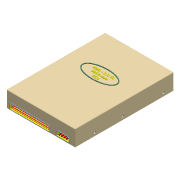
# Autodesk Inventor part: Hdd
Saved by Autodesk Inventor 2016 (Build 200138000, 138)
## iProperties
Created: 2017-12-22
Part Number: Hdd
Material: Generic
Document SubType Name: Modeling
Designer: Adrian
Density: 1 g/cm^3
Appearance: Dark Gray
Author: Adrian
Autodesk Inventor part; units mm, degrees
note: some values were not read from the file. Chosen so that the rebuilt part matches the saved one: offset side.
ref_plane "YZ Plane" through (0, 0, 0) normal (1, 0, 0) x (0, 1, 0)
ref_plane "XZ Plane" through (0, 0, 0) normal (0, 1, 0) x (-1, 0, 0)
ref_plane "XY Plane" through (0, 0, 0) normal (0, 0, 1) x (1, 0, 0)
sketch "Sketch1" plane through (0, 0, 0) normal (0, 0, 1) x (1, 0, 0)
  line L0 (-50.5, -72.5) -> (50.5, -72.5)
  line L1 (50.5, -72.5) -> (50.5, 72.5)
  line L2 (50.5, 72.5) -> (-50.5, 72.5)
  line L3 (-50.5, 72.5) -> (-50.5, -72.5)
  line L4 (0, 101.5) -> (0, -101.5) projected
  line L5 (-70.7, 0) -> (70.7, 0) projected
  dimension "d0" = 101
  dimension "d1" = 145
  dimension "d18" = 50.5
  dimension "d19" = 72.5
  constraints: 8 end point, 2 parallel, 1 horizontal, 1 perpendicular
  measures "d0" distance of L2.end L1.end
  measures "d1" distance of L1.end L0.end
  measures "d18" distance between parallel lines of L1 L4
  measures "d19" distance between parallel lines of L5 L2
extrude "Extrusion1" add sketch "Sketch1" along normal blind 24
fillet "Fillet1" radius 1 4 edges at (0, -72.5, 24) (50.5, 0, 24) (0, 72.5, 24) (-50.5, 0, 24)
fillet "Fillet2" radius 1 4 edges at (0, -72.5, 0) (-50.5, 0, 0) (0, 72.5, 0) (50.5, 0, 0)
fillet "Fillet3" radius 1 12 edges at (-50.2071, 72.2071, 23.7071) (-50.2071, 72.2071, 0.2929) (-50.5, 72.5, 12) (-50.2071, -72.2071, 23.7071) (-50.2071, -72.2071, 0.2929) (-50.5, -72.5, 12) (50.2071, -72.2071, 23.7071) (50.2071, -72.2071, 0.2929) (50.5, -72.5, 12) (50.2071, 72.2071, 23.7071) (50.2071, 72.2071, 0.2929) (50.5, 72.5, 12)
sketch "Sketch2" plane through (-50.5, -71.5, 23) normal (-1, 0, 0) x (0, 0, 1)
  line L0 (-23, 143) -> (-23, 0) projected
  line L1 (0, 144) -> (-22, 144) projected
  point P0 (-18, 129)
  point P1 (-18, 69)
  point P2 (-18, 28)
  dimension "d7" = 5
  dimension "d8" = 15
  dimension "d9" = 60
  dimension "d10" = 41
  constraints: 2 vertical alignment
  measures "d7" distance from line of L0 point (-18, 28)
  measures "d8" distance from line of L1 point (-18, 129)
  measures "d9" distance of point (-18, 129) point (-18, 69)
  measures "d10" distance of point (-18, 28) point (-18, 69)
hole "Hole1" at (-50.5, 57.5, 5) at (-50.5, -2.5, 5) at (-50.5, -43.5, 5) direction (1, 0, 0) diameter 3.242 depth 11.8 tip angle 118 thread size "M4x0.7" class "6H" standard "ISO Metric profile"
mirror "Mirror1" about plane through (0, 0, 0) normal (1, 0, 0) of "Hole1"
sketch "Sketch3" plane through (-49.5, -72.5, 23) normal (0, -1, 0) x (1, 0, 0)
  line L0 (4.4644, -13.9434) -> (62.4644, -13.9434)
  line L1 (62.4644, -13.9434) -> (62.4644, -20.9434)
  line L2 (62.4644, -20.9434) -> (4.4644, -20.9434)
  line L3 (4.4644, -20.9434) -> (4.4644, -13.9434)
  dimension "d20" = 7
  dimension "d21" = 58
  constraints: 8 end point, 2 parallel, 1 horizontal, 1 perpendicular
  measures "d20" distance of L2.end L0.start
  measures "d21" distance of L0.start L0.end
extrude "Extrusion2" cut sketch "Sketch3" against normal blind 8
sketch "Sketch4" plane through (-49.5, -64.5, 23) normal (0, -1, 0) x (1, 0, 0)
  line L0 (4.4644, -13.9434) -> (62.4644, -13.9434) projected
  line L1 (4.4644, -20.9434) -> (4.4644, -13.9434) projected
  circle A0 centre (7.0044, -16.4834) radius 0.5
  dimension "d26" = 2.54
  dimension "d27" = 2.54
  dimension "d34" = 1
  constraints: 1 centre point, 1 coincident
  measures "d26" distance from line of L0 point (7.004, -16.483)
  measures "d27" distance from line of L1 point (7.004, -16.483)
  measures "d34" diameter of A0
extrude "Extrusion3" add sketch "Sketch4" along normal blind 8
pattern_linear "Rectangular Pattern2" count 24 spacing 2.54 along (1, 0, 0) count 2 spacing 2.54 along (0, 0, -1) of "Extrusion3"
sketch "Sketch5" plane through (0, 0, 24) normal (0, 0, 1) x (1, 0, 0)
  line L0 (-19.8246, 19.2815) -> (19.8246, 19.2815) construction
  line L1 (19.8246, 19.2815) -> (19.8246, 9.0193) construction
  line L2 (19.8246, 9.0193) -> (-19.8246, 9.0193) construction
  line L3 (-19.8246, 9.0193) -> (-19.8246, 19.2815) construction
  line L4 (49.5, 72.5) -> (-49.5, 72.5) construction
  line L5 (-12.1323, 18.1219) -> (-13.0115, 18.1219)
  line L6 (-13.0115, 18.1219) -> (-13.0115, 19.6734)
  line L7 (-13.0115, 19.6734) -> (-14.2056, 19.6734)
  line L8 (-14.2056, 19.6734) -> (-14.2056, 18.1219)
  line L9 (-14.2056, 18.1219) -> (-15.0849, 18.1219)
  line L10 (-15.0849, 18.1219) -> (-15.0849, 21.6219)
  line L11 (-15.0849, 21.6219) -> (-14.2056, 21.6219)
  line L12 (-14.2056, 21.6219) -> (-14.2056, 20.3399)
  line L13 (-14.2056, 20.3399) -> (-13.0115, 20.3399)
  line L14 (-13.0115, 20.3399) -> (-13.0115, 21.6219)
  line L15 (-13.0115, 21.6219) -> (-12.1323, 21.6219)
  line L16 (-12.1323, 21.6219) -> (-12.1323, 18.1219)
  spline S0 degree 2 poles (-8.2834, 19.8691) (-8.2834, 19.3784) (-8.7117, 18.6069) (-9.0379, 18.3999) knots 0 0 0 1 2 2 2
  spline S1 degree 2 poles (-9.0379, 18.3999) (-9.3102, 18.224) (-9.9512, 18.1219) (-10.3114, 18.1219) knots 0 0 0 1 2 2 2
  line L17 (-10.3114, 18.1219) -> (-11.4062, 18.1219)
  line L18 (-11.4062, 18.1219) -> (-11.4062, 21.6219)
  line L19 (-11.4062, 21.6219) -> (-10.3227, 21.6219)
  spline S2 degree 2 poles (-10.3227, 21.6219) (-9.954, 21.6219) (-9.3102, 21.5283) (-9.0265, 21.3468) knots 0 0 0 1 2 2 2
  spline S3 degree 2 poles (-9.0265, 21.3468) (-8.6833, 21.1256) (-8.2834, 20.3768) (-8.2834, 19.8691) knots 0 0 0 1 2 2 2
  spline S4 degree 2 poles (-9.1854, 19.8747) (-9.1854, 20.2208) (-9.4236, 20.7143) (-9.6675, 20.8533) knots 0 0 0 1 2 2 2
  spline S5 degree 2 poles (-9.6675, 20.8533) (-9.8462, 20.9497) (-10.2376, 20.9696) (-10.5099, 20.9696) knots 0 0 0 1 2 2 2
  line L20 (-10.5099, 20.9696) -> (-10.5269, 20.9696)
  line L21 (-10.5269, 20.9696) -> (-10.5269, 18.7771)
  line L22 (-10.5269, 18.7771) -> (-10.5099, 18.7771)
  spline S6 degree 2 poles (-10.5099, 18.7771) (-10.215, 18.7771) (-9.8094, 18.7969) (-9.625, 18.9132) knots 0 0 0 1 2 2 2
  spline S7 degree 2 poles (-9.625, 18.9132) (-9.4094, 19.0494) (-9.1854, 19.5287) (-9.1854, 19.8747) knots 0 0 0 1 2 2 2
  spline S8 degree 2 poles (-4.6388, 19.8691) (-4.6388, 19.3784) (-5.0671, 18.6069) (-5.3932, 18.3999) knots 0 0 0 1 2 2 2
  spline S9 degree 2 poles (-5.3932, 18.3999) (-5.6655, 18.224) (-6.3065, 18.1219) (-6.6667, 18.1219) knots 0 0 0 1 2 2 2
  line L23 (-6.6667, 18.1219) -> (-7.7615, 18.1219)
  line L24 (-7.7615, 18.1219) -> (-7.7615, 21.6219)
  line L25 (-7.7615, 21.6219) -> (-6.6781, 21.6219)
  spline S10 degree 2 poles (-6.6781, 21.6219) (-6.3094, 21.6219) (-5.6655, 21.5283) (-5.3819, 21.3468) knots 0 0 0 1 2 2 2
  spline S11 degree 2 poles (-5.3819, 21.3468) (-5.0387, 21.1256) (-4.6388, 20.3768) (-4.6388, 19.8691) knots 0 0 0 1 2 2 2
  spline S12 degree 2 poles (-5.5407, 19.8747) (-5.5407, 20.2208) (-5.779, 20.7143) (-6.0229, 20.8533) knots 0 0 0 1 2 2 2
  spline S13 degree 2 poles (-6.0229, 20.8533) (-6.2016, 20.9497) (-6.593, 20.9696) (-6.8653, 20.9696) knots 0 0 0 1 2 2 2
  line L26 (-6.8653, 20.9696) -> (-6.8823, 20.9696)
  line L27 (-6.8823, 20.9696) -> (-6.8823, 18.7771)
  line L28 (-6.8823, 18.7771) -> (-6.8653, 18.7771)
  spline S14 degree 2 poles (-6.8653, 18.7771) (-6.5703, 18.7771) (-6.1647, 18.7969) (-5.9803, 18.9132) knots 0 0 0 1 2 2 2
  spline S15 degree 2 poles (-5.9803, 18.9132) (-5.7648, 19.0494) (-5.5407, 19.5287) (-5.5407, 19.8747) knots 0 0 0 1 2 2 2
  line L29 (-1.2551, 19.3415) -> (-2.8122, 19.3415)
  line L30 (-2.8122, 19.3415) -> (-2.8122, 19.9939)
  line L31 (-2.8122, 19.9939) -> (-1.2551, 19.9939)
  line L32 (-1.2551, 19.9939) -> (-1.2551, 19.3415)
  line L33 (3.1866, 18.1219) -> (0.875, 18.1219)
  line L34 (0.875, 18.1219) -> (0.875, 18.7317)
  line L35 (0.875, 18.7317) -> (1.6124, 18.7317)
  line L36 (1.6124, 18.7317) -> (1.6124, 20.5838)
  line L37 (1.6124, 20.5838) -> (0.875, 20.5838)
  line L38 (0.875, 20.5838) -> (0.875, 21.1539)
  spline S16 degree 2 poles (0.875, 21.1539) (1.0367, 21.1539) (1.3572, 21.1965) (1.4536, 21.2418) knots 0 0 0 1 2 2 2
  spline S17 degree 2 poles (1.4536, 21.2418) (1.5642, 21.2986) (1.689, 21.4886) (1.7004, 21.6304) knots 0 0 0 1 2 2 2
  line L39 (1.7004, 21.6304) -> (2.4662, 21.6304)
  line L40 (2.4662, 21.6304) -> (2.4662, 18.7317)
  line L41 (2.4662, 18.7317) -> (3.1866, 18.7317)
  line L42 (3.1866, 18.7317) -> (3.1866, 18.1219)
  line L43 (4.6473, 18.1219) -> (3.8162, 18.1219)
  line L44 (3.8162, 18.1219) -> (3.8162, 19.0465)
  line L45 (3.8162, 19.0465) -> (4.6473, 19.0465)
  line L46 (4.6473, 19.0465) -> (4.6473, 18.1219)
  spline S18 degree 2 poles (7.8665, 19.8719) (7.8665, 19.4181) (7.7218, 18.7374) (7.5602, 18.5076) knots 0 0 0 1 2 2 2
  spline S19 degree 2 poles (7.5602, 18.5076) (7.4013, 18.2807) (6.888, 18.0482) (6.5192, 18.0482) knots 0 0 0 1 2 2 2
  spline S20 degree 2 poles (6.5192, 18.0482) (6.1477, 18.0482) (5.6372, 18.2807) (5.4755, 18.5133) knots 0 0 0 1 2 2 2
  spline S21 degree 2 poles (5.4755, 18.5133) (5.3138, 18.7431) (5.1692, 19.4181) (5.1692, 19.8719) knots 0 0 0 1 2 2 2
  spline S22 degree 2 poles (5.1692, 19.8719) (5.1692, 20.3371) (5.3138, 20.9951) (5.4783, 21.2333) knots 0 0 0 1 2 2 2
  spline S23 degree 2 poles (5.4783, 21.2333) (5.6428, 21.4659) (6.1619, 21.6928) (6.5192, 21.6928) knots 0 0 0 1 2 2 2
  spline S24 degree 2 poles (6.5192, 21.6928) (6.8965, 21.6928) (7.4013, 21.4546) (7.563, 21.2192) knots 0 0 0 1 2 2 2
  spline S25 degree 2 poles (7.563, 21.2192) (7.7218, 20.9894) (7.8665, 20.3115) (7.8665, 19.8719) knots 0 0 0 1 2 2 2
  spline S26 degree 2 poles (6.9844, 19.8719) (6.9844, 20.5214) (6.7717, 21.0461) (6.5192, 21.0461) knots 0 0 0 1 2 2 2
  spline S27 degree 2 poles (6.5192, 21.0461) (6.2668, 21.0461) (6.0513, 20.5214) (6.0513, 19.8691) knots 0 0 0 1 2 2 2
  spline S28 degree 2 poles (6.0513, 19.8691) (6.0513, 19.2281) (6.2668, 18.6948) (6.5192, 18.6948) knots 0 0 0 1 2 2 2
  spline S29 degree 2 poles (6.5192, 18.6948) (6.7688, 18.6948) (6.9844, 19.2281) (6.9844, 19.8719) knots 0 0 0 1 2 2 2
  line L47 (10.4957, 18.1219) -> (10.4957, 20.9554)
  line L48 (10.4957, 20.9554) -> (9.4605, 20.9554)
  line L49 (9.4605, 20.9554) -> (9.4605, 21.6219)
  line L50 (9.4605, 21.6219) -> (12.4103, 21.6219)
  line L51 (12.4103, 21.6219) -> (12.4103, 20.9554)
  line L52 (12.4103, 20.9554) -> (11.375, 20.9554)
  line L53 (11.375, 20.9554) -> (11.375, 18.1219)
  line L54 (11.375, 18.1219) -> (10.4957, 18.1219)
  spline S30 degree 2 poles (15.309, 19.4777) (15.309, 18.848) (14.6708, 18.0709) (14.1971, 18.0709) knots 0 0 0 1 2 2 2
  spline S31 degree 2 poles (14.1971, 18.0709) (14.0014, 18.0709) (13.7093, 18.1588) (13.5448, 18.2524) knots 0 0 0 1 2 2 2
  line L55 (13.5448, 18.2524) -> (13.5107, 18.1219)
  line L56 (13.5107, 18.1219) -> (12.7222, 18.1219)
  line L57 (12.7222, 18.1219) -> (12.7222, 21.7779)
  line L58 (12.7222, 21.7779) -> (13.5448, 21.7779)
  line L59 (13.5448, 21.7779) -> (13.5448, 20.4845)
  spline S32 degree 2 poles (13.5448, 20.4845) (13.7263, 20.6405) (14.1007, 20.8334) (14.3474, 20.8334) knots 0 0 0 1 2 2 2
  spline S33 degree 2 poles (14.3474, 20.8334) (14.8098, 20.8334) (15.309, 20.1158) (15.309, 19.4777) knots 0 0 0 1 2 2 2
  spline S34 degree 2 poles (14.4666, 19.4606) (14.4666, 19.8549) (14.2283, 20.1924) (13.9787, 20.1924) knots 0 0 0 1 2 2 2
  spline S35 degree 2 poles (13.9787, 20.1924) (13.8681, 20.1924) (13.6497, 20.1215) (13.5448, 20.0506) knots 0 0 0 1 2 2 2
  line L60 (13.5448, 20.0506) -> (13.5448, 18.7289)
  spline S36 degree 2 poles (13.5448, 18.7289) (13.627, 18.6948) (13.7944, 18.6721) (13.8766, 18.6721) knots 0 0 0 1 2 2 2
  spline S37 degree 2 poles (13.8766, 18.6721) (14.1744, 18.6721) (14.4666, 19.0664) (14.4666, 19.4606) knots 0 0 0 1 2 2 2
  line L61 (-8.8393, 15.1644) -> (-10.3341, 12.3592)
  line L62 (-10.3341, 12.3592) -> (-11.3098, 12.3592)
  line L63 (-11.3098, 12.3592) -> (-9.747, 15.1984)
  line L64 (-9.747, 15.1984) -> (-11.4147, 15.1984)
  line L65 (-11.4147, 15.1984) -> (-11.4147, 15.8592)
  line L66 (-11.4147, 15.8592) -> (-8.8393, 15.8592)
  line L67 (-8.8393, 15.8592) -> (-8.8393, 15.1644)
  line L68 (-5.6967, 12.3592) -> (-8.2692, 12.3592)
  line L69 (-8.2692, 12.3592) -> (-8.2692, 12.9293)
  spline S38 degree 2 poles (-8.2692, 12.9293) (-7.9431, 13.1903) (-7.4212, 13.6498) (-7.2255, 13.8568) knots 0 0 0 1 2 2 2
  spline S39 degree 2 poles (-7.2255, 13.8568) (-6.9674, 14.1263) (-6.7376, 14.5375) (-6.7376, 14.7531) knots 0 0 0 1 2 2 2
  spline S40 degree 2 poles (-6.7376, 14.7531) (-6.7376, 14.997) (-7.0298, 15.258) (-7.2907, 15.258) knots 0 0 0 1 2 2 2
  spline S41 degree 2 poles (-7.2907, 15.258) (-7.424, 15.258) (-7.6623, 15.1927) (-7.7842, 15.1417) knots 0 0 0 1 2 2 2
  spline S42 degree 2 poles (-7.7842, 15.1417) (-7.9034, 15.0878) (-8.0735, 14.9743) (-8.1161, 14.946) knots 0 0 0 1 2 2 2
  line L70 (-8.1161, 14.946) -> (-8.1842, 14.946)
  line L71 (-8.1842, 14.946) -> (-8.1842, 15.7089)
  spline S43 degree 2 poles (-8.1842, 15.7089) (-8.0367, 15.7798) (-7.407, 15.9273) (-7.1149, 15.9273) knots 0 0 0 1 2 2 2
  spline S44 degree 2 poles (-7.1149, 15.9273) (-6.4909, 15.9273) (-5.8499, 15.3714) (-5.8499, 14.8694) knots 0 0 0 1 2 2 2
  spline S45 degree 2 poles (-5.8499, 14.8694) (-5.8499, 14.5602) (-6.142, 13.9646) (-6.4795, 13.6242) knots 0 0 0 1 2 2 2
  spline S46 degree 2 poles (-6.4795, 13.6242) (-6.6923, 13.4144) (-7.0922, 13.0882) (-7.1801, 13.0201) knots 0 0 0 1 2 2 2
  line L72 (-7.1801, 13.0201) -> (-5.6967, 13.0201)
  line L73 (-5.6967, 13.0201) -> (-5.6967, 12.3592)
  spline S47 degree 2 poles (-2.6761, 14.1092) (-2.6761, 13.6554) (-2.8207, 12.9747) (-2.9824, 12.745) knots 0 0 0 1 2 2 2
  spline S48 degree 2 poles (-2.9824, 12.745) (-3.1412, 12.5181) (-3.6546, 12.2855) (-4.0233, 12.2855) knots 0 0 0 1 2 2 2
  spline S49 degree 2 poles (-4.0233, 12.2855) (-4.3949, 12.2855) (-4.9054, 12.5181) (-5.0671, 12.7507) knots 0 0 0 1 2 2 2
  spline S50 degree 2 poles (-5.0671, 12.7507) (-5.2287, 12.9804) (-5.3734, 13.6554) (-5.3734, 14.1092) knots 0 0 0 1 2 2 2
  spline S51 degree 2 poles (-5.3734, 14.1092) (-5.3734, 14.5744) (-5.2287, 15.2324) (-5.0642, 15.4707) knots 0 0 0 1 2 2 2
  spline S52 degree 2 poles (-5.0642, 15.4707) (-4.8997, 15.7033) (-4.3807, 15.9302) (-4.0233, 15.9302) knots 0 0 0 1 2 2 2
  spline S53 degree 2 poles (-4.0233, 15.9302) (-3.6461, 15.9302) (-3.1412, 15.6919) (-2.9795, 15.4565) knots 0 0 0 1 2 2 2
  spline S54 degree 2 poles (-2.9795, 15.4565) (-2.8207, 15.2268) (-2.6761, 14.5489) (-2.6761, 14.1092) knots 0 0 0 1 2 2 2
  spline S55 degree 2 poles (-3.5581, 14.1092) (-3.5581, 14.7588) (-3.7709, 15.2835) (-4.0233, 15.2835) knots 0 0 0 1 2 2 2
  spline S56 degree 2 poles (-4.0233, 15.2835) (-4.2757, 15.2835) (-4.4913, 14.7588) (-4.4913, 14.1064) knots 0 0 0 1 2 2 2
  spline S57 degree 2 poles (-4.4913, 14.1064) (-4.4913, 13.4654) (-4.2757, 12.9322) (-4.0233, 12.9322) knots 0 0 0 1 2 2 2
  spline S58 degree 2 poles (-4.0233, 12.9322) (-3.7737, 12.9322) (-3.5581, 13.4654) (-3.5581, 14.1092) knots 0 0 0 1 2 2 2
  spline S59 degree 2 poles (0.39, 14.1092) (0.39, 13.6554) (0.2453, 12.9747) (0.0837, 12.745) knots 0 0 0 1 2 2 2
  spline S60 degree 2 poles (0.0837, 12.745) (-0.0752, 12.5181) (-0.5885, 12.2855) (-0.9573, 12.2855) knots 0 0 0 1 2 2 2
  spline S61 degree 2 poles (-0.9573, 12.2855) (-1.3288, 12.2855) (-1.8393, 12.5181) (-2.001, 12.7507) knots 0 0 0 1 2 2 2
  spline S62 degree 2 poles (-2.001, 12.7507) (-2.1627, 12.9804) (-2.3073, 13.6554) (-2.3073, 14.1092) knots 0 0 0 1 2 2 2
  spline S63 degree 2 poles (-2.3073, 14.1092) (-2.3073, 14.5744) (-2.1627, 15.2324) (-1.9982, 15.4707) knots 0 0 0 1 2 2 2
  spline S64 degree 2 poles (-1.9982, 15.4707) (-1.8337, 15.7033) (-1.3146, 15.9302) (-0.9573, 15.9302) knots 0 0 0 1 2 2 2
  spline S65 degree 2 poles (-0.9573, 15.9302) (-0.58, 15.9302) (-0.0752, 15.6919) (0.0865, 15.4565) knots 0 0 0 1 2 2 2
  spline S66 degree 2 poles (0.0865, 15.4565) (0.2453, 15.2268) (0.39, 14.5489) (0.39, 14.1092) knots 0 0 0 1 2 2 2
  spline S67 degree 2 poles (-0.4921, 14.1092) (-0.4921, 14.7588) (-0.7048, 15.2835) (-0.9573, 15.2835) knots 0 0 0 1 2 2 2
  spline S68 degree 2 poles (-0.9573, 15.2835) (-1.2097, 15.2835) (-1.4252, 14.7588) (-1.4252, 14.1064) knots 0 0 0 1 2 2 2
  spline S69 degree 2 poles (-1.4252, 14.1064) (-1.4252, 13.4654) (-1.2097, 12.9322) (-0.9573, 12.9322) knots 0 0 0 1 2 2 2
  spline S70 degree 2 poles (-0.9573, 12.9322) (-0.7077, 12.9322) (-0.4921, 13.4654) (-0.4921, 14.1092) knots 0 0 0 1 2 2 2
  line L74 (4.0715, 14.2199) -> (4.0034, 14.2199)
  spline S71 degree 2 poles (4.0034, 14.2199) (3.9552, 14.2369) (3.7765, 14.2539) (3.6688, 14.2539) knots 0 0 0 1 2 2 2
  spline S72 degree 2 poles (3.6688, 14.2539) (3.5411, 14.2539) (3.2547, 14.1773) (3.1214, 14.1263) knots 0 0 0 1 2 2 2
  line L75 (3.1214, 14.1263) -> (3.1214, 12.3592)
  line L76 (3.1214, 12.3592) -> (2.2988, 12.3592)
  line L77 (2.2988, 12.3592) -> (2.2988, 14.9998)
  line L78 (2.2988, 14.9998) -> (3.1214, 14.9998)
  line L79 (3.1214, 14.9998) -> (3.1214, 14.6198)
  spline S73 degree 2 poles (3.1214, 14.6198) (3.1781, 14.6708) (3.3766, 14.8297) (3.4589, 14.8779) knots 0 0 0 1 2 2 2
  spline S74 degree 2 poles (3.4589, 14.8779) (3.5496, 14.9318) (3.7879, 15.0084) (3.8928, 15.0084) knots 0 0 0 1 2 2 2
  spline S75 degree 2 poles (3.8928, 15.0084) (3.9325, 15.0084) (4.0318, 15.0027) (4.0715, 14.9998) knots 0 0 0 1 2 2 2
  line L80 (4.0715, 14.9998) -> (4.0715, 14.2199)
  spline S76 degree 2 poles (6.9731, 13.715) (6.9731, 13.0825) (6.332, 12.3082) (5.8612, 12.3082) knots 0 0 0 1 2 2 2
  spline S77 degree 2 poles (5.8612, 12.3082) (5.6655, 12.3082) (5.3734, 12.3961) (5.2089, 12.4926) knots 0 0 0 1 2 2 2
  line L81 (5.2089, 12.4926) -> (5.2089, 11.3921)
  line L82 (5.2089, 11.3921) -> (4.3863, 11.3921)
  line L83 (4.3863, 11.3921) -> (4.3863, 14.9998)
  line L84 (4.3863, 14.9998) -> (5.2089, 14.9998)
  line L85 (5.2089, 14.9998) -> (5.2089, 14.7219)
  spline S78 degree 2 poles (5.2089, 14.7219) (5.3904, 14.8779) (5.7648, 15.0708) (6.0115, 15.0708) knots 0 0 0 1 2 2 2
  spline S79 degree 2 poles (6.0115, 15.0708) (6.471, 15.0708) (6.9731, 14.3418) (6.9731, 13.715) knots 0 0 0 1 2 2 2
  spline S80 degree 2 poles (6.1307, 13.698) (6.1307, 14.0837) (5.8924, 14.4298) (5.6428, 14.4298) knots 0 0 0 1 2 2 2
  spline S81 degree 2 poles (5.6428, 14.4298) (5.5322, 14.4298) (5.3138, 14.3588) (5.2089, 14.2879) knots 0 0 0 1 2 2 2
  line L86 (5.2089, 14.2879) -> (5.2089, 12.9634)
  spline S82 degree 2 poles (5.2089, 12.9634) (5.2741, 12.935) (5.4329, 12.9123) (5.5407, 12.9123) knots 0 0 0 1 2 2 2
  spline S83 degree 2 poles (5.5407, 12.9123) (5.8385, 12.9123) (6.1307, 13.3037) (6.1307, 13.698) knots 0 0 0 1 2 2 2
  line L87 (10.5667, 12.3592) -> (10.5667, 13.6781)
  spline S84 degree 2 poles (10.5667, 13.6781) (10.5667, 13.8738) (10.5525, 14.1404) (10.5184, 14.2255) knots 0 0 0 1 2 2 2
  spline S85 degree 2 poles (10.5184, 14.2255) (10.4816, 14.3106) (10.3341, 14.3872) (10.2008, 14.3872) knots 0 0 0 1 2 2 2
  spline S86 degree 2 poles (10.2008, 14.3872) (10.1072, 14.3872) (9.9256, 14.305) (9.8179, 14.2284) knots 0 0 0 1 2 2 2
  line L88 (9.8179, 14.2284) -> (9.8179, 12.3592)
  line L89 (9.8179, 12.3592) -> (8.9897, 12.3592)
  line L90 (8.9897, 12.3592) -> (8.9897, 13.6781)
  spline S87 degree 2 poles (8.9897, 13.6781) (8.9897, 13.871) (8.9726, 14.1404) (8.9386, 14.2255) knots 0 0 0 1 2 2 2
  spline S88 degree 2 poles (8.9386, 14.2255) (8.9017, 14.3106) (8.7543, 14.3872) (8.6209, 14.3872) knots 0 0 0 1 2 2 2
  spline S89 degree 2 poles (8.6209, 14.3872) (8.5217, 14.3872) (8.326, 14.2936) (8.2352, 14.2284) knots 0 0 0 1 2 2 2
  line L91 (8.2352, 14.2284) -> (8.2352, 12.3592)
  line L92 (8.2352, 12.3592) -> (7.4127, 12.3592)
  line L93 (7.4127, 12.3592) -> (7.4127, 14.9998)
  line L94 (7.4127, 14.9998) -> (8.2352, 14.9998)
  line L95 (8.2352, 14.9998) -> (8.2352, 14.7077)
  spline S90 degree 2 poles (8.2352, 14.7077) (8.4366, 14.8779) (8.7968, 15.0708) (9.0209, 15.0708) knots 0 0 0 1 2 2 2
  spline S91 degree 2 poles (9.0209, 15.0708) (9.262, 15.0708) (9.6307, 14.841) (9.7271, 14.6113) knots 0 0 0 1 2 2 2
  spline S92 degree 2 poles (9.7271, 14.6113) (9.9625, 14.8325) (10.3823, 15.0708) (10.5979, 15.0708) knots 0 0 0 1 2 2 2
  spline S93 degree 2 poles (10.5979, 15.0708) (10.7822, 15.0708) (11.0744, 14.9545) (11.1736, 14.8353) knots 0 0 0 1 2 2 2
  spline S94 degree 2 poles (11.1736, 14.8353) (11.2842, 14.7077) (11.3949, 14.3588) (11.3949, 14.078) knots 0 0 0 1 2 2 2
  line L96 (11.3949, 14.078) -> (11.3949, 12.3592)
  line L97 (11.3949, 12.3592) -> (10.5667, 12.3592)
  spline S95 degree 2 poles (-2.9994, 6.5228) (-3.7056, 6.5228) (-4.4658, 7.2036) (-4.4658, 7.8616) knots 0 0 0 1 2 2 2
  line L98 (-4.4658, 7.8616) -> (-4.4658, 10.0966)
  line L99 (-4.4658, 10.0966) -> (-3.5865, 10.0966)
  line L100 (-3.5865, 10.0966) -> (-3.5865, 7.9126)
  spline S96 degree 2 poles (-3.5865, 7.9126) (-3.5865, 7.5468) (-3.3114, 7.1894) (-2.9994, 7.1894) knots 0 0 0 1 2 2 2
  spline S97 degree 2 poles (-2.9994, 7.1894) (-2.6959, 7.1894) (-2.4123, 7.5326) (-2.4123, 7.9126) knots 0 0 0 1 2 2 2
  line L101 (-2.4123, 7.9126) -> (-2.4123, 10.0966)
  line L102 (-2.4123, 10.0966) -> (-1.533, 10.0966)
  line L103 (-1.533, 10.0966) -> (-1.533, 7.8644)
  spline S98 degree 2 poles (-1.533, 7.8644) (-1.533, 7.2177) (-2.2733, 6.5228) (-2.9994, 6.5228) knots 0 0 0 1 2 2 2
  spline S99 degree 2 poles (0.6509, 6.5285) (-0.1376, 6.5285) (-1.0622, 7.4815) (-1.0622, 8.3438) knots 0 0 0 1 2 2 2
  spline S100 degree 2 poles (-1.0622, 8.3438) (-1.0622, 9.1748) (-0.1347, 10.1647) (0.6538, 10.1647) knots 0 0 0 1 2 2 2
  spline S101 degree 2 poles (0.6538, 10.1647) (0.8608, 10.1647) (1.1955, 10.1164) (1.3487, 10.0767) knots 0 0 0 1 2 2 2
  spline S102 degree 2 poles (1.3487, 10.0767) (1.4678, 10.0399) (1.7486, 9.9179) (1.8365, 9.8725) knots 0 0 0 1 2 2 2
  line L104 (1.8365, 9.8725) -> (1.8365, 9.0386)
  line L105 (1.8365, 9.0386) -> (1.7486, 9.0386)
  spline S103 degree 2 poles (1.7486, 9.0386) (1.6833, 9.0954) (1.4905, 9.2542) (1.3685, 9.328) knots 0 0 0 1 2 2 2
  spline S104 degree 2 poles (1.3685, 9.328) (1.2466, 9.4045) (0.9544, 9.5095) (0.7927, 9.5095) knots 0 0 0 1 2 2 2
  spline S105 degree 2 poles (0.7927, 9.5095) (0.6027, 9.5095) (0.2879, 9.3904) (0.1432, 9.24) knots 0 0 0 1 2 2 2
  spline S106 degree 2 poles (0.1432, 9.24) (0.0128, 9.1067) (-0.1546, 8.6501) (-0.1546, 8.3409) knots 0 0 0 1 2 2 2
  spline S107 degree 2 poles (-0.1546, 8.3409) (-0.1546, 8.0147) (0.0184, 7.5694) (0.1603, 7.4333) knots 0 0 0 1 2 2 2
  spline S108 degree 2 poles (0.1603, 7.4333) (0.2964, 7.3) (0.6311, 7.1837) (0.7984, 7.1837) knots 0 0 0 1 2 2 2
  spline S109 degree 2 poles (0.7984, 7.1837) (0.9714, 7.1837) (1.2863, 7.3) (1.394, 7.3709) knots 0 0 0 1 2 2 2
  spline S110 degree 2 poles (1.394, 7.3709) (1.5132, 7.4418) (1.6919, 7.5921) (1.7571, 7.6517) knots 0 0 0 1 2 2 2
  line L106 (1.7571, 7.6517) -> (1.8365, 7.6517)
  line L107 (1.8365, 7.6517) -> (1.8365, 6.8292)
  spline S111 degree 2 poles (1.8365, 6.8292) (1.7401, 6.7838) (1.4876, 6.6703) (1.3515, 6.6306) knots 0 0 0 1 2 2 2
  spline S112 degree 2 poles (1.3515, 6.6306) (1.187, 6.5796) (0.9005, 6.5285) (0.6509, 6.5285) knots 0 0 0 1 2 2 2
  line L108 (4.7778, 9.2372) -> (3.8304, 6.5966)
  line L109 (3.8304, 6.5966) -> (2.9313, 6.5966)
  line L110 (2.9313, 6.5966) -> (1.9925, 9.2372)
  line L111 (1.9925, 9.2372) -> (2.8576, 9.2372)
  line L112 (2.8576, 9.2372) -> (3.3965, 7.4929)
  line L113 (3.3965, 7.4929) -> (3.9297, 9.2372)
  line L114 (3.9297, 9.2372) -> (4.7778, 9.2372)
  point P0 (0, 19.2815)
  point P1 (0, 72.5)
  constraints: 2 midpoint, 1 vertical alignment, 2 other
sketch "Sketch6" plane through (-49.5, -72.5, 23) normal (0, -1, 0) x (1, 0, 0)
  line L0 (73, -16.5) -> (73, -20.5)
  line L1 (73, -20.5) -> (91, -20.5)
  line L2 (91, -20.5) -> (91, -16.5)
  line L3 (91, -16.5) -> (89, -14.5)
  line L4 (89, -14.5) -> (75, -14.5)
  line L5 (75, -14.5) -> (73, -16.5)
  line L6 (0, -23) -> (99, -23) projected
  line L7 (100, -22) -> (100, 0) projected
  dimension "d43" = 18
  dimension "d44" = 6
  dimension "d45" = 2.5
  dimension "d46" = 9
  dimension "d47" = 14
  constraints: 12 end point, 3 perpendicular, 2 equal length, 1 parallel, 1 vertical
  measures "d43" distance of L0.end L1.end
  measures "d44" distance between parallel lines of L1 L4
  measures "d45" distance between parallel lines of L6 L1
  measures "d46" distance between parallel lines of L7 L2
  measures "d47" distance of L3.end L4.end
extrude "Extrusion4" cut sketch "Sketch6" against normal blind 8
sketch "Sketch7" plane through (-49.5, -64.5, 23) normal (0, -1, 0) x (1, 0, 0)
  circle A0 centre (76.5, -18.1) radius 1
  line L0 (91, -20.5) -> (73, -20.5) projected
  circle A1 centre (80, -18.1) radius 1
  circle A2 centre (83.5, -18.1) radius 1
  circle A3 centre (87, -18.1) radius 1
  line L1 (73, -20.5) -> (73, -16.5) projected
  dimension "d50" = 2
  dimension "d51" = 2.4
  dimension "d52" = 2
  dimension "d53" = 2
  dimension "d54" = 2
  dimension "d55" = 3.5
  dimension "d56" = 3.5
  dimension "d57" = 3.5
  dimension "d58" = 3.5
  constraints: 4 centre point, 3 horizontal alignment
  measures "d50" diameter of A0
  measures "d51" distance from line of A0.centre L0
  measures "d52" diameter of A1
  measures "d53" diameter of A2
  measures "d54" diameter of A3
  measures "d55" distance of A1.centre A0.centre
  measures "d56" distance of A2.centre A1.centre
  measures "d57" distance of A2.centre A3.centre
  measures "d58" distance from line of L1 A0.centre
extrude "Extrusion5" add sketch "Sketch7" along normal blind 8
emboss "Emboss1" sketch "Sketch5" operation add depth 0.5 direction (0, 0, -1)
sketch "Sketch8" plane through (0, 0, 24) normal (0, 0, 1) x (1, 0, 0)
  ellipse E0 centre (-0.9531, 15.131) end of major axis (23.6816, 15.131) minor radius 11
  spline S0 degree 5 poles (24.9651, 15.131) (24.9653, 16.1313) (24.7625, 17.1354) (24.3584, 18.0741) (23.186, 19.9455) (21.5488, 21.4383) (20.5863, 22.1466) (18.3248, 23.5487) (15.8809, 24.6052) (14.5028, 25.1059) (11.4979, 26.0258) (8.4178, 26.6535) (6.7611, 26.9162) (3.3532, 27.3167) (-0.0758, 27.4483) (-1.8306, 27.4483) (-5.2595, 27.3167) (-8.6674, 26.9161) (-10.324, 26.6535) (-13.4041, 26.0258) (-16.4089, 25.106) (-17.7871, 24.6052) (-20.231, 23.5489) (-22.4927, 22.1464) (-23.4552, 21.4387) (-25.0925, 19.9447) (-26.2646, 18.0748) (-26.669, 17.1336) (-27.0739, 15.131) (-26.669, 13.1283) (-26.2646, 12.1872) (-25.0925, 10.3173) (-23.4552, 8.8233) (-22.4927, 8.1155) (-20.231, 6.713) (-17.7871, 5.6568) (-16.4089, 5.1559) (-13.4041, 4.2362) (-10.324, 3.6084) (-8.6674, 3.3458) (-5.2595, 2.9452) (-1.8306, 2.8136) (-0.0758, 2.8136) (3.3532, 2.9452) (6.7611, 3.3458) (8.4178, 3.6085) (11.4979, 4.2361) (14.5028, 5.156) (15.8809, 5.6567) (18.3248, 6.7133) (20.5863, 8.1153) (21.5488, 8.8236) (23.186, 10.3165) (24.3584, 12.1878) (24.7625, 13.1266) (24.9653, 14.1306) (24.9651, 15.131) knots 0 0 0 0 0 0 0.04031 0.04031 0.04031 0.088263 0.088263 0.088263 0.147213 0.147213 0.147213 0.214697 0.214697 0.214697 0.285304 0.285304 0.285304 0.352786 0.352786 0.352786 0.411736 0.411736 0.411736 0.459692 0.459692 0.459692 0.5 0.5 0.5 0.540308 0.540308 0.540308 0.588264 0.588264 0.588264 0.647214 0.647214 0.647214 0.714696 0.714696 0.714696 0.785303 0.785303 0.785303 0.852787 0.852787 0.852787 0.911737 0.911737 0.911737 0.95969 0.95969 0.95969 1 1 1 1 1 1
  dimension "d69" = 11
  constraints: 2 other
extrude "Extrusion6" add sketch "Sketch8" along normal blind 0.5
sketch "Sketch9" plane through (-49.5, -72.5, 23) normal (0, -1, 0) x (1, 0, 0)
  line L0 (4.4644, -13.9434) -> (62.4644, -13.9434) projected
  line L1 (4.4644, -20.9434) -> (4.4644, -13.9434) projected
  line L2 (62.4644, -20.9434) -> (4.4644, -20.9434) projected
  line L3 (62.4644, -13.9434) -> (62.4644, -16.2121) projected
  line L4 (62.4644, -19.2946) -> (62.4644, -20.9434) projected
  line L5 (73, -20.5) -> (73, -16.5) projected
  line L6 (73, -16.5) -> (75, -14.5) projected
  line L7 (75, -14.5) -> (89, -14.5) projected
  line L8 (89, -14.5) -> (91, -16.5) projected
  line L9 (91, -16.5) -> (91, -20.5) projected
  circle A0 centre (83.5, -18.1) radius 1 projected
  circle A1 centre (76.5, -18.1) radius 1 projected
  circle A2 centre (80, -18.1) radius 1 projected
  circle A3 centre (87, -18.1) radius 1 projected
  line L10 (73, -20.5) -> (73, -16.5) projected
  line L11 (91, -20.5) -> (73, -20.5) projected
  line L12 (91, -16.5) -> (91, -20.5) projected
  line L13 (89, -14.5) -> (91, -16.5) projected
  line L14 (75, -14.5) -> (89, -14.5) projected
  line L15 (73, -16.5) -> (75, -14.5) projected
  line L16 (72, -21.5) -> (72, -16.0858)
  line L17 (72, -16.0858) -> (74.5858, -13.5)
  line L18 (74.5858, -13.5) -> (89.4142, -13.5)
  line L19 (89.4142, -13.5) -> (92, -16.0858)
  line L20 (92, -16.0858) -> (92, -21.5)
  line L21 (92, -21.5) -> (72, -21.5)
  line L22 (63.4644, -16.2121) -> (63.4644, -12.9434)
  line L23 (63.4644, -12.9434) -> (3.4644, -12.9434)
  line L24 (3.4644, -12.9434) -> (3.4644, -21.9434)
  line L25 (3.4644, -21.9434) -> (63.4644, -21.9434)
  line L26 (63.4644, -21.9434) -> (63.4644, -19.2946)
  line L27 (63.4644, -16.2121) -> (63.4644, -19.2946)
  line L28 (62.4644, -19.2946) -> (62.4644, -16.2121)
  dimension "d65" = 1
  dimension "d66" = 1
  constraints: 26 end point, 2 vertical, 9 other
  measures "d65" distance between parallel lines of L0 L23
  measures "d66" distance between parallel lines of L18 L7
extrude "Extrusion7" add sketch "Sketch9" along normal blind 0.5 contours L16 L17 L18 L19 L20 L21 | L27 L26 L25 L24 L23 L22
equation "\"d18\" = 0.5 * d0"
equation "\"d19\" = 0.5 * d1"
equation "\"d52\" = d50"
equation "\"d53\" = d50"
equation "\"d54\" = d50"
equation "\"d56\" = d55"
equation "\"d57\" = d55"
body "Solid1"
